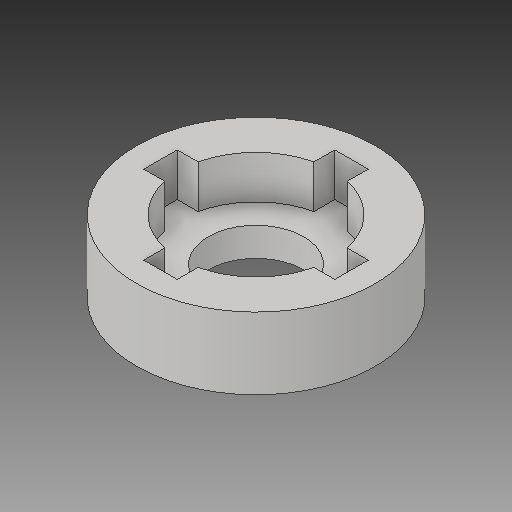
# Autodesk Inventor part: adapter
Saved by Autodesk Inventor 2019.3 (Build 233278000, 278)
## iProperties
Created: 2020-01-24
Part Number: adapter
Material: Generisch
Document SubType Name: Modeling
Designer: 9frick
Density: 1 g/cm^3
Appearance: Vorgabe
Mass: 19.2889 g
Surface Area: 72.5048 cm^2
Volume: 19.2889 cm^3
Author: 9frick
Autodesk Inventor part; units mm, degrees
ref_plane "YZ Plane" through (0, 0, 0) normal (1, 0, 0) x (0, 1, 0)
ref_plane "XZ Plane" through (0, 0, 0) normal (0, 1, 0) x (-1, 0, 0)
ref_plane "XY Plane" through (0, 0, 0) normal (0, 0, 1) x (1, 0, 0)
sketch "Sketch1" plane through (0, 0, 0) normal (0, 1, 0) x (-1, 0, 0)
  circle A0 centre (0, 0) radius 25
  circle A1 centre (0, 0) radius 10
  dimension "d0" = 50
  dimension "d1" = 20
  constraints: 2 centre point, 2 coincident
  measures "d0" diameter of A0
  measures "d1" diameter of A1
extrude "Extrusion1" add sketch "Sketch1" along normal blind 15
sketch "Sketch2" plane through (0, 15, 0) normal (0, 1, 0) x (1, 0, 0)
  line L0 (20, 0) -> (20, -3.5)
  line L1 (20, -3.5) -> (15.6125, -3.5)
  line L2 (-20, -3.5) -> (-20, 3.5)
  line L3 (20, 3.5) -> (20, -3.5)
  line L4 (-20, 3.5) -> (-15.6125, 3.5)
  line L5 (15.6125, 3.5) -> (20, 3.5)
  line L6 (20, -3.5) -> (15.6125, -3.5)
  line L7 (-15.6125, -3.5) -> (-20, -3.5)
  line L8 (0, 20) -> (3.5, 20)
  line L9 (3.5, 20) -> (3.5, 15.6125)
  line L10 (3.5, -20) -> (-3.5, -20)
  line L11 (-3.5, 20) -> (3.5, 20)
  line L12 (-3.5, -20) -> (-3.5, -15.6125)
  line L13 (-3.5, 15.6125) -> (-3.5, 20)
  line L14 (3.5, 20) -> (3.5, 15.6125)
  line L15 (3.5, -15.6125) -> (3.5, -20)
  line L16 (0, 20) -> (3.5, 20)
  line L17 (3.5, 20) -> (3.5, 15.6125)
  line L18 (3.5, -20) -> (-3.5, -20)
  line L19 (-3.5, 20) -> (3.5, 20)
  line L20 (-3.5, -20) -> (-3.5, -15.6125)
  line L21 (-3.5, 15.6125) -> (-3.5, 20)
  line L22 (3.5, 20) -> (3.5, 15.6125)
  line L23 (3.5, -15.6125) -> (3.5, -20)
  arc A0 (15.6125, 3.5) -> (3.5, 15.6125) centre (0, 0) ccw
  arc A1 (-3.5, 15.6125) -> (-15.6125, 3.5) centre (0, 0) ccw
  arc A2 (-3.5, 15.6125) -> (-15.6125, 3.5) centre (0, 0) ccw
  arc A3 (-15.6125, -3.5) -> (-3.5, -15.6125) centre (0, 0) ccw
  arc A4 (-15.6125, -3.5) -> (-3.5, -15.6125) centre (0, 0) ccw
  arc A5 (3.5, -15.6125) -> (15.6125, -3.5) centre (0, 0) ccw
  arc A6 (-3.5, 15.6125) -> (-15.6125, 3.5) centre (0, 0) ccw
  arc A7 (-15.6125, -3.5) -> (-3.5, -15.6125) centre (0, 0) ccw
  arc A8 (3.5, -15.6125) -> (15.6125, -3.5) centre (0, 0) ccw
  arc A9 (15.6125, 3.5) -> (3.5, 15.6125) centre (0, 0) ccw
  arc A10 (3.5, -15.6125) -> (15.6125, -3.5) centre (0, 0) ccw
  arc A11 (15.6125, 3.5) -> (3.5, 15.6125) centre (0, 0) ccw
  dimension "d7" = 40
  dimension "d8" = 7
  constraints: 48 end point, 24 point on circle, 15 parallel, 12 centre point, 6 perpendicular, 2 horizontal, 1 coincident
  measures "d7" distance of L2.end L3.start
  measures "d8" distance of L2.start L2.end
extrude "Extrusion2" cut sketch "Sketch2" against normal blind 9
body "Solid1"
